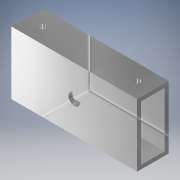
# Autodesk Inventor part: 15102898-16-P-0306
Saved by Autodesk Inventor 2017 (Build 210142000, 142)
## iProperties
Created: 2016-10-05
Part Number: 15102898-16-P-0306
Material: Aluminum 6061
Document SubType Name: Modeling
Designer: 15102898
Density: 2.7 g/cm^3
Appearance: Aluminum - Flat
Author: 15102898
Autodesk Inventor part; units mm, degrees
ref_plane "YZ Plane" through (0, 0, 0) normal (1, 0, 0) x (0, 1, 0)
ref_plane "XZ Plane" through (0, 0, 0) normal (0, 1, 0) x (-1, 0, 0)
ref_plane "XY Plane" through (0, 0, 0) normal (0, 0, 1) x (1, 0, 0)
sketch "Sketch1" plane through (0, 0, 0) normal (0, 1, 0) x (-1, 0, 0)
  line L0 (0, 0) -> (101.6, 0)
  line L1 (101.6, 0) -> (101.6, 25.4)
  line L2 (101.6, 25.4) -> (0, 25.4)
  line L3 (0, 25.4) -> (0, 0)
  dimension "d0" = 101.6
  dimension "d1" = 25.4
  constraints: 8 end point, 2 parallel, 1 horizontal, 1 perpendicular
  measures "d0" distance of L1.end L2.end
  measures "d1" distance of L2.end L0.start
extrude "Extrusion1" add sketch "Sketch1" along normal blind 50.8
sketch "Sketch2" plane through (-101.6, 0, 25.4) normal (0, 0, 1) x (1, 0, 0)
  circle A0 centre (25.4, 19.05) radius 7.9375
  line L0 (101.6, 50.8) -> (0, 50.8) projected
  line L1 (101.6, 0) -> (101.6, 50.8) projected
  dimension "d4" = 15.875
  dimension "d5" = 31.75
  dimension "d6" = 76.2
  constraints: 1 centre point
  measures "d4" diameter of A0
  measures "d5" distance from line of L0 A0.centre
  measures "d6" distance from line of L1 A0.centre
extrude "Extrusion2" cut sketch "Sketch2" against normal blind 111.125
sketch "Sketch3" plane through (0, 0, 25.4) normal (1, 0, 0) x (0, 0, -1)
  line L0 (3.175, 3.175) -> (22.225, 3.175)
  line L1 (22.225, 3.175) -> (22.225, 47.625)
  line L2 (22.225, 47.625) -> (3.175, 47.625)
  line L3 (3.175, 47.625) -> (3.175, 3.175)
  line L4 (0, 0) -> (0, 50.8) projected
  line L5 (0, 0) -> (25.4, 0) projected
  line L6 (25.4, 0) -> (25.4, 50.8) projected
  line L7 (25.4, 50.8) -> (0, 50.8) projected
  dimension "d9" = 3.175
  dimension "d10" = 3.175
  dimension "d11" = 3.175
  dimension "d12" = 3.175
  constraints: 8 end point, 2 parallel, 1 horizontal, 1 perpendicular
  measures "d9" distance between parallel lines of L4 L3
  measures "d10" distance between parallel lines of L5 L0
  measures "d11" distance between parallel lines of L6 L1
  measures "d12" distance between parallel lines of L7 L2
extrude "Extrusion3" cut sketch "Sketch3" against normal blind 111.125 contours L3 L2 L1 L0
sketch "Sketch4" plane through (0, 50.8, 0) normal (0, 1, 0) x (1, 0, 0)
  circle A0 centre (-12.7, -12.827) radius 2.54
  circle A1 centre (-88.9, -12.827) radius 2.54
  line L0 (0, 0) -> (-101.6, 0) projected
  line L1 (-101.6, 0) -> (-101.6, -25.4) projected
  line L2 (0, -25.4) -> (0, 0) projected
  dimension "d15" = 5.08
  dimension "d16" = 12.827
  dimension "d17" = 12.7
  dimension "d18" = 5.08
  dimension "d19" = 12.827
  dimension "d20" = 12.7
  dimension "d21" = 76.2
  constraints: 2 centre point
  measures "d15" diameter of A1
  measures "d16" distance from line of L0 A1.centre
  measures "d17" distance from line of L1 A1.centre
  measures "d18" diameter of A0
  measures "d19" distance from line of L0 A0.centre
  measures "d20" distance from line of L2 A0.centre
  measures "d21" distance of A0.centre A1.centre
extrude "Extrusion4" cut sketch "Sketch4" against normal blind 111.125
sketch "Sketch5" plane through (-101.6, 0, 25.4) normal (0, 0, 1) x (1, 0, 0)
  circle A0 centre (25.4, 19.05) radius 7.9375 projected
  circle A1 centre (25.4, 19.05) radius 14.2875
  point P0 (101.6, 0)
  dimension "d24" = 28.575
  constraints: 1 centre point, 1 coincident
  measures "d24" diameter of A1
extrude "Extrusion5" cut sketch "Sketch5" against normal blind 5.08
body "Solid1"
